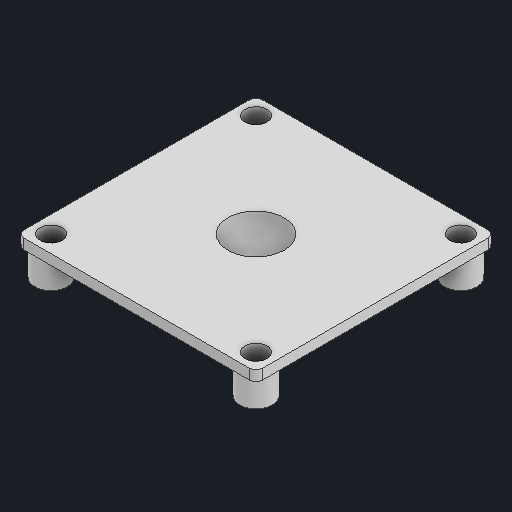
# Autodesk Inventor part: cradle_holder_with_septa
Saved by Autodesk Inventor 2025 (Build 290162010, 162A)
## iProperties
Created: 2024-06-21
Part Number: cradle_holder_with_septa
Material: Generic
Document SubType Name: Modeling
Designer: mihir
Density: 1 g/cm^3
Appearance: Default
Author: mihir
Autodesk Inventor part; units mm, degrees
ref_plane "YZ Plane" through (0, 0, 0) normal (1, 0, 0) x (0, 1, 0)
ref_plane "XZ Plane" through (0, 0, 0) normal (0, 1, 0) x (-1, 0, 0)
ref_plane "XY Plane" through (0, 0, 0) normal (0, 0, 1) x (1, 0, 0)
sketch "Sketch1" plane through (0, 0, 0) normal (0, 1, 0) x (-1, 0, 0)
  line L0 (0, 0) -> (70, 0)
  line L1 (70, 0) -> (70, -70)
  line L2 (70, -70) -> (0, -70)
  line L3 (0, -70) -> (0, 0)
  circle A0 centre (5, -5) radius 3.25
  circle A1 centre (5, -65) radius 3.25
  circle A2 centre (65, -5) radius 3.25
  circle A3 centre (65, -65) radius 3.25
  dimension "d0" = 70
  dimension "d1" = 6.5
  dimension "d4" = 60
  dimension "d7" = 60
  dimension "d10" = 5
  dimension "d11" = 5
  constraints: 8 end point, 4 centre point, 2 horizontal, 2 parallel, 2 perpendicular, 1 vertical, 6 other
  measures "d0" distance of L2.end L0.start
  measures "d1" diameter of A0
  measures "d4" distance of A0.centre A1.centre
  measures "d7" distance of A0.centre A2.centre
  measures "d10" distance from line of L3 A0.centre
  measures "d11" distance from line of L0 A0.centre
extrude "Extrusion1" add sketch "Sketch1" along normal blind 3
fillet "Fillet1" radius 2 4 edges at (-70, 1.5, 0) (-70, 1.5, -70) (0, 1.5, -70) (0, 1.5, 0)
sketch "Sketch2" plane through (0, 3, 0) normal (0, 1, 0) x (1, 0, 0)
  line L0 (-70, 68) -> (-70, 2) construction
  line L1 (-70, 35) -> (0, 35) construction
  line L2 (0, 2) -> (0, 68) construction
  line L3 (-68, 0) -> (-2, 0) construction
  line L4 (-35, 0) -> (-35, 70) construction
  line L5 (-2, 70) -> (-68, 70) construction
  arc A0 (-35, 43.25) -> (-35, 26.75) centre (-35, 35) ccw
  arc A1 (-35, 46.25) -> (-35, 23.75) centre (-35, 35) ccw
  line L6 (-35, 23.75) -> (-35, 26.75)
  line L7 (-35, 43.25) -> (-35, 46.25)
  point P0 (0, 0)
  dimension "d17" = 8.25
  dimension "d19" = 3
  constraints: 8 end point, 5 midpoint, 4 point on circle, 4 point on line, 2 centre point, 1 coincident, 1 vertical
  measures "d17" radius of A0
  measures "d19" radial gap between concentric circles of A0 A1
revolve "Revolution1" add sketch "Sketch2" angle 180 about axis through (-35, 3, 0) along (0, 0, 1)
sketch "Sketch3" plane through (0, 3, 0) normal (0, 1, 0) x (1, 0, 0)
  circle A0 centre (-35, 35) radius 8.25
  circle A1 centre (-35, 35) radius 7.6852 projected
  line L0 (-43.25, 35) -> (-26.75, 35)
  point P0 (0, 0)
  point P1 (-42.6852, 35)
  point P2 (-27.3148, 35)
  dimension "d40" = 16.5
  constraints: 2 end point, 2 point on circle, 1 centre point, 1 concentric, 1 horizontal, 1 midpoint
  measures "d40" diameter of A0
revolve "Revolution2" cut sketch "Sketch3" angle 180 about axis through (-43.25, 3, -35) along (-1, 0, 0) picked at (-42.9818, 35.6581) picked at (-32.6573, 36.8036) contours L0 A1 A0 | L0 A1
sketch "Sketch4" plane through (0, 3, 0) normal (0, 1, 0) x (1, 0, 0)
  circle A0 centre (-35, 35) radius 7.6852 projected
  point P0 (0, 0)
  constraints: 1 coincident
hole "Hole1" at (-35, 3, -35) direction (0, -1, 0) diameter 3 end through all
sketch "Sketch5" plane through (0, 0, 0) normal (0, -1, 0) x (1, 0, 0)
  circle A0 centre (-5, -5) radius 3.25 projected
  circle A1 centre (-5, -5) radius 4.775
  circle A2 centre (-5, -5) radius 3.25
  line L0 (-68, 0) -> (-2, 0) projected
  line L1 (0, -2) -> (0, -68) projected
  circle A3 centre (-65, -5) radius 4.775
  circle A4 centre (-65, -5) radius 3.25
  circle A5 centre (-5, -65) radius 4.775
  circle A6 centre (-5, -65) radius 3.25
  circle A7 centre (-65, -65) radius 4.775
  circle A8 centre (-65, -65) radius 3.25
  point P0 (0, 0)
  dimension "d29" = 9.55
  dimension "d32" = 60
  dimension "d35" = 60
  constraints: 8 centre point, 2 coincident, 1 concentric, 1 horizontal, 1 vertical, 12 other
  measures "d29" diameter of A1
  measures "d32" distance of A1.centre A3.centre
  measures "d35" distance of A1.centre A5.centre
extrude "Extrusion2" add sketch "Sketch5" along normal blind 8
equation "\"d0\" = cradle_width"
equation "\"d1\" = rod_diameter + rod_free_tolerance"
equation "\"d4\" = rod_dist"
equation "\"d7\" = rod_dist"
equation "\"d10\" = 0.5 * cradle_width - 0.5 * rod_dist"
equation "\"d11\" = 0.5 * cradle_width - 0.5 * rod_dist"
equation "\"d12\" = cradle_holder_thickness"
equation "\"d17\" = 0.5 * tube_diameter"
equation "\"d19\" = cradle_holder_thickness"
equation "\"d40\" = tube_diameter"
equation "\"d22\" = needle_hole_diameter"
equation "\"d29\" = post_diameter - post_wall_diameter"
equation "\"d32\" = rod_dist"
equation "\"d35\" = rod_dist"
equation "\"d38\" = cradle_holder_peg_depth"
equation "\"cradle_width\" = 70"
equation "\"cradle_holder_peg_depth\" = 8"
equation "\"tube_diameter\" = 16.5"
equation "\"rod_dist\" = 60"
equation "\"rod_diameter\" = 6"
equation "\"rod_free_tolerance\" = 0.5"
equation "\"cradle_holder_thickness\" = 3"
equation "\"needle_hole_diameter\" = 3"
equation "\"post_diameter\" = 10.2"
equation "\"post_wall_diameter\" = 0.65"
body "Solid1"
